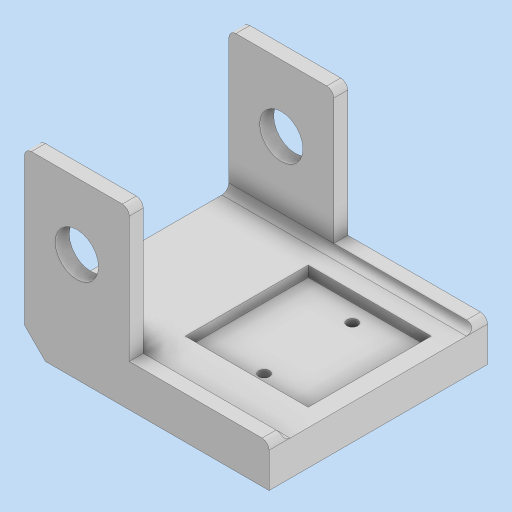
# Autodesk Inventor part: base_engrane
Saved by Autodesk Inventor 2024 (Build 280153000, 153)
## iProperties
Created: 2024-09-04
Part Number: base_engrane
Material: Generic
Document SubType Name: Modeling
Designer: MxMon
Density: 1 g/cm^3
Appearance: Default
Author: MxMon
Autodesk Inventor part; units mm, degrees
ref_plane "YZ Plane" through (0, 0, 0) normal (1, 0, 0) x (0, 1, 0)
sketch "Sketch1" plane through (0, 0, 0) normal (0, 1, 0) x (-1, 0, 0)
  line L0 (20, 31.25) -> (-20, 31.25)
  line L1 (-20, 31.25) -> (-20, -31.25)
  line L2 (-20, -31.25) -> (20, -31.25)
  line L3 (20, -31.25) -> (20, 31.25)
  line L4 (20, 31.25) -> (-20, -31.25) construction
  line L5 (-20, 31.25) -> (20, -31.25) construction
  point P0 (0, 0)
  dimension "d0" = 40
  dimension "d1" = 62.5
  constraints: 12 end point, 2 midpoint, 2 parallel, 1 horizontal, 1 perpendicular
  measures "d0" distance of L2.end L1.end
  measures "d1" distance of L1.end L0.end
extrude "Extrusion1" add sketch "Sketch1" along normal blind 50
sketch "Sketch2" plane through (0, 50, 0) normal (0, 1, 0) x (1, 0, 0)
  line L0 (20, -31.25) -> (20, 31.25) projected
  line L1 (-20, -27.25) -> (20, -27.25)
  line L2 (20, -27.25) -> (20, 27.25)
  line L3 (20, 27.25) -> (-20, 27.25)
  line L4 (-20, 27.25) -> (-20, -27.25)
  line L5 (-20, -27.25) -> (20, 27.25) construction
  line L6 (20, -27.25) -> (-20, 27.25) construction
  line L7 (-20, -31.25) -> (20, -31.25) projected
  point P0 (0, 0)
  dimension "d4" = 4
  constraints: 12 end point, 2 midpoint, 2 parallel, 1 horizontal, 1 perpendicular, 1 point on line
  measures "d4" distance between parallel lines of L7 L1
extrude "Extrusion2" cut sketch "Sketch2" against normal blind 40
sketch "Sketch3" plane through (-20, 0, 31.25) normal (0, 0, 1) x (1, 0, 0)
  circle A0 centre (15, 31) radius 6.2
  line L0 (40, 10) -> (0, 10) projected
  line L1 (40, 10) -> (40, 50) projected
  line L2 (0, 0) -> (0, 50) projected
  point P0 (20, 0)
  point P1 (40, 30)
  dimension "d7" = 12.4
  dimension "d15" = 21
  dimension "d38" = 15
  constraints: 1 centre point, 1 midpoint
  measures "d7" diameter of A0
  measures "d15" vertical distance of L0.start A0.centre
  measures "d38" distance from line of L2 A0.centre
extrude "Extrusion3" cut sketch "Sketch3" against normal blind 8
sketch "Sketch4" plane through (20, 0, -31.25) normal (0, 0, -1) x (-1, 0, 0)
  circle A0 centre (25, 31) radius 6.2 projected
  point P0 (20, 0)
extrude "Extrusion4" cut sketch "Sketch4" against normal blind 8
fillet "Fillet1" radius 2 2 edges at (0, 10, 27.25) (0, 10, -27.25)
sketch "Sketch5" plane through (20, 0, 31.25) normal (1, 0, 0) x (0, 0, -1)
  line L0 (4, 12) -> (4, 50) projected
  line L1 (0, 50) -> (4, 50) projected
  line L2 (0, 0) -> (0, 50) projected
  arc A0 (4, 12) -> (6, 10) centre (6, 12) ccw projected
  line L3 (0, 0) -> (62.5, 0) projected
  line L4 (56.5, 10) -> (6, 10) projected
  arc A1 (56.5, 10) -> (58.5, 12) centre (56.5, 12) ccw projected
  line L5 (58.5, 50) -> (58.5, 12) projected
  line L6 (62.5, 0) -> (62.5, 50) projected
  line L7 (58.5, 50) -> (62.5, 50) projected
  point P0 (31.25, 0)
extrude "Extrusion5" add sketch "Sketch5" along normal blind 30
sketch "Sketch6" plane through (0, 10, 0) normal (0, 1, 0) x (1, 0, 0)
  line L0 (9.748, 20.2) -> (44.948, 20.2)
  line L1 (44.948, 20.2) -> (44.948, -15)
  line L2 (44.948, -15) -> (9.748, -15)
  line L3 (9.748, -15) -> (9.748, 20.2)
  line L4 (9.748, 20.2) -> (44.948, -15) construction
  line L5 (44.948, 20.2) -> (9.748, -15) construction
  line L6 (-20, -25.25) -> (-20, 25.25) projected
  point P0 (0, 0)
  point P1 (27.348, 2.6)
  point P2 (-20, 0)
  point P3 (44.948, 2.6)
  dimension "d16" = 35.2
  dimension "d17" = 35.2
  dimension "d18" = 65
  dimension "d84" = 2.6
  constraints: 12 end point, 4 midpoint, 2 parallel, 1 horizontal, 1 perpendicular
  measures "d16" distance of L1.end L2.end
  measures "d17" distance of L0.end L1.end
  measures "d18" distance of point (-20, 0) point (44.948, 2.6)
  measures "d84" vertical distance of point (0, 0) point (27.348, 2.6)
extrude "Extrusion6" cut sketch "Sketch6" against normal blind 3
sketch "Sketch10" plane through (0, 0, 0) normal (0, -1, 0) x (1, 0, 0)
  line L0 (44.948, 15) -> (9.748, 15) projected
  line L1 (44.948, -20.2) -> (44.948, 15) projected
  line L2 (9.748, -20.2) -> (44.948, -20.2) projected
  line L3 (9.748, 15) -> (9.748, -20.2) projected
  point P0 (0, 0)
  point P1 (27.348, -15.2)
  point P2 (27.348, -20.2)
  dimension "d37" = 5
  constraints: 1 midpoint, 1 vertical alignment
  measures "d37" distance from line of point (27.348, -15.2) L2
hole "Hole1" at (27.348, 0, -15.2) direction (0, 1, 0) diameter 3.1 end through all countersink diameter 4 countersink angle 90
ref_plane "Work Plane1" through (20, 0, -31.25) normal (-1, 0, 0) x (0, 0, 1)
fillet "Fillet4" radius 2 4 edges at (-20, 50, -29.25) (50, 50, -29.25) (50, 50, 29.25) (-20, 50, 29.25)
sketch "Sketch16" plane through (50, 0, -31.25) normal (0, 0, -1) x (-1, 0, 0)
  line L0 (68, 50) -> (2, 50) projected
  arc A0 (2, 50) -> (0, 48) centre (2, 48) ccw projected
  line L1 (0, 0) -> (0, 48) projected
  line L2 (0, 12) -> (70, 12) projected
  line L3 (40, 50) -> (40, 12)
  point P0 (50, 0)
  dimension "d93" = 40
  constraints: 2 end point, 2 point on line
  measures "d93" distance between parallel lines of L1 L3
extrude "Extrusion14" cut sketch "Sketch16" against normal blind 4
fillet "Fillet5" radius 2 1 edges at (10, 50, -29.25)
sketch "Sketch17" plane through (-20, 0, 31.25) normal (0, 0, 1) x (1, 0, 0)
  line L0 (2, 50) -> (68, 50) projected
  line L1 (70, 48) -> (70, 0) projected
  arc A0 (70, 48) -> (68, 50) centre (68, 48) ccw projected
  line L2 (0, 12) -> (70, 12) projected
  line L3 (30, 50) -> (30, 12)
  point P0 (20, 0)
  dimension "d88" = 40
  constraints: 2 end point, 2 point on line, 1 vertical
  measures "d88" distance between parallel lines of L1 L3
extrude "Extrusion15" cut sketch "Sketch17" against normal blind 4
fillet "Fillet6" radius 2 2 edges at (50, 12, 29.25) (50, 12, -29.25)
fillet "Fillet7" radius 2 1 edges at (10, 50, 29.25)
ref_plane "Work Plane2" through (44.948, 10, -2.6) normal (0, 0, -1) x (-1, 0, 0)
mirror "Mirror5" about plane through (44.948, 10, -2.6) normal (0, 0, -1) of "Hole1"
chamfer "Chamfer1" distance 6 angle 45 1 edges at (-20, 0, 0)
body "Solid1"
